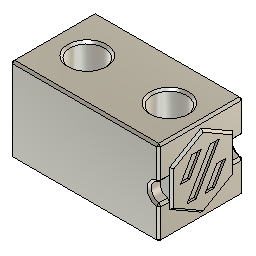
Fystec M5 Insert Nut Block v7 (Autodesk Fusion 360 design; units mm, degrees)
Autodesk Fusion 360 part; units mm, degrees
sketch "Sketch1" plane through (0, 0, 0) normal (0, 0, 1) x (1, 0, 0)
  line L0 (0, 0) -> (28, 0)
  line L1 (28, 0) -> (28, 16)
  line L2 (28, 16) -> (0, 16)
  line L3 (0, 16) -> (0, 0)
  dimension "d1" = 28
  dimension "d2" = 16
  constraint horizontal L0
  constraint vertical L1
  constraint horizontal L2
  constraint vertical L3
  constraint coincident L0.start L3.end
  measures "d1" distance of L0.start L0.end
  measures "d2" distance of L0.start L2.end
extrude "Extrude1" add sketch "Sketch1" along normal blind 16
sketch "Sketch2" plane through (0, 0, 16) normal (0, 0, 1) x (-1, 0, 0)
  line L0 (0, -16) -> (0, 0)
  line L1 (0, 0) -> (-28, 0)
  line L2 (-28, 0) -> (-28, -16)
  line L3 (-28, -16) -> (0, -16)
  line L4 (0, -8) -> (-28, -8) construction
  line L5 (-6.5, -16) -> (-6.5, 0) construction
  line L6 (-22, -16) -> (-22, 0) construction
  circle A0 centre (-6.5, -8) radius 3.25
  circle A1 centre (-22, -8) radius 3.25
  dimension "d5" = 6.5
  dimension "d6" = 15.5
  dimension "d7" = 6.5
  dimension "d8" = 6.5
  constraint midpoint L0 L4.start
  constraint midpoint L2 L4.end
  constraint coincident L3 L5.start
  constraint coincident L1 L5.end
  constraint perpendicular L1 L5
  constraint coincident L3 L6.start
  constraint coincident L1 L6.end
  constraint perpendicular L1 L6
  constraint midpoint L5 A0.centre
  constraint midpoint L6 A1.centre
  measures "d5" distance of L0 L5
  measures "d6" distance of L5 L6
  measures "d7" diameter of A0
  measures "d8" diameter of A1
extrude "Extrude2" cut sketch "Sketch2" against normal blind 6 contours A0 | A1
sketch "Sketch3" plane through (0, 0, 0) normal (0, 0, -1) x (1, 0, 0)
  line L0 (0, 0) -> (0, -16)
  line L1 (0, -16) -> (28, -16)
  line L2 (28, -16) -> (28, 0)
  line L3 (28, 0) -> (0, 0)
  circle A0 centre (6.5, -8) radius 3.25
  circle A1 centre (22, -8) radius 3.25
extrude "Extrude3" cut sketch "Sketch3" against normal blind 6 contours A0 | A1
sketch "Sketch4" plane through (28, 0, 0) normal (1, 0, 0) x (0, 1, 0)
  line L0 (0, 0) -> (16, 0)
  line L1 (16, 0) -> (16, 16)
  line L2 (16, 16) -> (0, 16)
  line L3 (0, 16) -> (0, 0)
  line L4 (7.6128, 11.7945) -> (5.4221, 8)
  line L5 (12.2966, 8) -> (10.1058, 4.2055)
  line L6 (2.0465, 11.4373) -> (8, 14.8745)
  line L7 (5.8942, 11.7945) -> (7.6128, 11.7945)
  line L8 (3.7034, 8) -> (5.8942, 11.7945)
  line L9 (9.3314, 11.7945) -> (4.95, 4.2055)
  line L10 (13.9535, 11.4373) -> (13.9535, 4.5627)
  line L11 (6.6686, 4.2055) -> (11.05, 11.7945)
  line L12 (10.5779, 8) -> (12.2966, 8)
  line L13 (8, 14.8745) -> (13.9535, 11.4373)
  line L14 (8, 1.1255) -> (2.0465, 4.5627)
  line L15 (2.0465, 4.5627) -> (2.0465, 11.4373)
  line L16 (8.3872, 4.2055) -> (10.5779, 8)
  line L17 (5.4221, 8) -> (3.7034, 8)
  line L18 (4.95, 4.2055) -> (6.6686, 4.2055)
  line L19 (11.05, 11.7945) -> (9.3314, 11.7945)
  line L20 (10.1058, 4.2055) -> (8.3872, 4.2055)
  line L21 (13.9535, 4.5627) -> (8, 1.1255)
  line L22 (7.0257, 8) -> (8.9743, 8) construction
  line L23 (0, 8) -> (16, 8) construction
  line L24 (8, 16) -> (8, 0) construction
  point P0 (8, 8)
  point P1 (8, 8)
  constraint horizontal L22
  constraint midpoint L3 L23.start
  constraint midpoint L1 L23.end
  constraint midpoint L2 L24.start
  constraint midpoint L0 L24.end
  constraint midpoint L22 P1
  constraint midpoint L24 P1
extrude "Extrude4" add sketch "Sketch4" along normal blind 0.4 contours L6 L10 L13 L14 L15 L21
sketch "Sketch5" plane through (0, 0, 0) normal (0, -1, 0) x (1, 0, 0)
  line L0 (0, 0) -> (28, 0)
  line L1 (28, 0) -> (28, 16)
  line L2 (28, 16) -> (0, 16)
  line L3 (0, 16) -> (0, 0)
  arc A0 (28, 9.8) -> (28, 6.2) centre (28, 8) ccw
  dimension "d25" = 1.8
  constraint midpoint L1 A0.centre
  measures "d25" radius of A0
sketch "Sketch6" plane through (0, 16, 0) normal (0, 1, 0) x (-1, 0, 0)
  line L0 (-28, 0) -> (0, 0)
  line L1 (0, 0) -> (0, 16)
  line L2 (0, 16) -> (-28, 16)
  line L3 (-28, 16) -> (-28, 0)
  arc A0 (-28, 6.2) -> (-28, 9.8) centre (-28, 8) ccw
extrude "Extrude8" cut sketch "Sketch5" against normal blind 2.0465 contours L1 A0
extrude "Extrude9" cut sketch "Sketch6" against normal blind 2.047 contours L3 A0
chamfer "Chamfer1" distance 0.4 angle 45 20 edges at (14, 0, 16) (28, 8, 16) (28, 0, 3.1) (28, 0, 12.9) (28, 16, 3.1) (28, 16, 12.9) (14, 16, 16) (0, 8, 16) (0, 16, 8) (14, 16, 0) (14, 0, 0) (0, 8, 0) (0, 0, 8) (28, 8, 0) (26.2, 0, 8) (28, 1.0232, 6.2) (28, 1.0232, 9.8) (26.2, 16, 8) (28, 14.9768, 6.2) (28, 14.9768, 9.8)
chamfer "Chamfer2" distance 0.4 angle 45 6 edges at (28.4, 5.0233, 13.1559) (28.4, 10.9768, 13.1559) (28.4, 2.0465, 8) (28.4, 5.0232, 2.8441) (28.4, 10.9768, 2.8441) (28.4, 13.9535, 8)
chamfer "Chamfer3" distance 0.4 angle 45 4 edges at (9.5301, 6.8247, 16) (25.0301, 6.8247, 16) (3.4699, 6.8247, 0) (18.9699, 6.8247, 0)
chamfer "Chamfer4" distance 0.6 angle 45 4 edges at (25.0301, 6.8247, 10) (9.5301, 6.8247, 10) (18.9699, 6.8247, 6) (3.4699, 6.8247, 6)
extrude "Extrude7" cut 2 faces at (7.0507, 8.6906, 10) (23.3948, 7.2286, 10) along direction (0, 0, -1) blind 4
